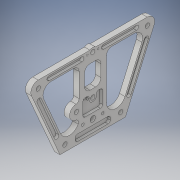
# Autodesk Inventor part: Frame_Bearing
Saved by Autodesk Inventor 2019 (Build 230136000, 136)
## iProperties
Created: 2019-07-29
Part Number: Frame_Bearing
Material: Generic
Document SubType Name: Modeling
Designer: 19879326
Density: 1 g/cm^3
Appearance: Default
Author: 19879326
Autodesk Inventor part; units mm, degrees
ref_plane "YZ Plane" through (0, 0, 0) normal (1, 0, 0) x (0, 1, 0)
ref_plane "XZ Plane" through (0, 0, 0) normal (0, 1, 0) x (-1, 0, 0)
ref_plane "XY Plane" through (0, 0, 0) normal (0, 0, 1) x (1, 0, 0)
sketch "Sketch1" plane through (0, 0, 0) normal (1, 0, 0) x (0, 1, 0)
  line L0 (73.575, 28) -> (65.075, 28)
  line L1 (-73.575, 60) -> (-73.575, -60)
  line L2 (73.575, -28) -> (73.575, 28)
  circle A0 centre (59.575, 0) radius 4
  circle A1 centre (-12.425, 0) radius 4
  circle A2 centre (-46.575, 0) radius 5
  circle A3 centre (-46.575, 18.25) radius 2.5
  circle A4 centre (-46.575, -18.25) radius 2.5
  circle A5 centre (59.575, 0) radius 7.5
  line L3 (65.075, 28) -> (65.075, 5.099)
  line L4 (65.075, -5.099) -> (65.075, -28)
  circle A6 centre (51.575, -100) radius 4
  circle A7 centre (51.575, 100) radius 4
  arc A8 (65.075, 100) -> (46.1655, 112.3688) centre (51.575, 100) ccw
  arc A9 (46.1655, -112.3688) -> (65.075, -100) centre (51.575, -100) ccw
  line L5 (65.075, 28) -> (65.075, 100)
  line L6 (65.075, -28) -> (65.075, -100)
  line L7 (46.1655, 112.3688) -> (-73.575, 60)
  line L8 (-73.575, -60) -> (46.1655, -112.3688)
  line L9 (65.075, -28) -> (73.575, -28)
  line L10 (30.0644, 90.0466) -> (-40.7048, 59.0955)
  line L11 (30.0644, -90.0466) -> (-40.7048, -59.0955)
  line L12 (51.075, 76.3035) -> (51.075, 35)
  line L13 (51.075, -76.3035) -> (51.075, -35)
  line L14 (41.075, 25) -> (-33.575, 25)
  line L15 (41.075, -25) -> (-33.575, -25)
  arc A10 (41.075, 25) -> (51.075, 35) centre (41.075, 35) ccw
  arc A11 (-40.7048, 59.0955) -> (-33.575, 25) centre (-33.575, 42.7932) ccw
  arc A12 (51.075, -35) -> (41.075, -25) centre (41.075, -35) ccw
  line L16 (-31.8814, -25) -> (-33.575, -25)
  arc A13 (-33.575, -25) -> (-40.7048, -59.0955) centre (-33.575, -42.7932) ccw
  line L17 (1.575, 5) -> (1.575, -5)
  arc A14 (43.575, 5) -> (33.575, 15) centre (33.575, 5) ccw
  arc A15 (33.575, -15) -> (43.575, -5) centre (33.575, -5) ccw
  arc A16 (11.575, 15) -> (1.575, 5) centre (11.575, 5) ccw
  arc A17 (1.575, -5) -> (11.575, -15) centre (11.575, -5) ccw
  circle A18 centre (-61.575, 51.0593) radius 4
  circle A19 centre (-61.575, -51.0593) radius 4
  arc A20 (51.075, 76.3035) -> (30.0644, 90.0466) centre (36.075, 76.3035) ccw
  arc A21 (30.0644, -90.0466) -> (51.075, -76.3035) centre (36.075, -76.3035) ccw
  line L18 (43.575, 5) -> (43.575, -5)
  line L19 (33.575, 15) -> (11.575, 15)
  line L20 (33.575, -15) -> (11.575, -15)
  circle A22 centre (-20.425, 30) radius 4
  circle A23 centre (-20.425, 30) radius 12.5
  point P0 (0, 0)
  point P1 (73.575, 0)
  point P2 (51.075, 58.5072)
  point P3 (51.075, -58.5072)
  point P4 (-20.425, -42.5)
  point P5 (16.0532, -25)
  point P6 (-49.2726, -25)
  point P7 (51.075, 59.4738)
  point P8 (43.575, 0)
  point P9 (1.575, 0)
  dimension "d1" = 56
  dimension "d2" = 72
  dimension "d3" = 8
  dimension "d4" = 8
  dimension "d5" = 14
  dimension "d6" = 34.15
  dimension "d7" = 10
  dimension "d8" = 18.25
  dimension "d9" = 18.25
  dimension "d10" = 5
  dimension "d13" = 12.425
  dimension "d14" = 27
  dimension "d15" = 15
  dimension "d18" = 5.5
  dimension "d19" = 8
  dimension "d20" = 100
  dimension "d21" = 100
  dimension "d22" = 8
  dimension "d27" = 60
  dimension "d28" = 60
  dimension "d31" = 14
  dimension "d33" = 14
  dimension "d34" = 14
  dimension "d36" = 25
  dimension "d37" = 25
  dimension "d43" = 40
  dimension "d45" = 14
  dimension "d47" = 12
  dimension "d48" = 13
  dimension "d49" = 13
  dimension "d50" = 12
  dimension "d58" = 10
  dimension "d59" = 15
  dimension "d60" = 16
  dimension "d61" = 10
  dimension "d62" = 10
  dimension "d90" = 8
  dimension "d91" = 25
  dimension "d92" = 30
  dimension "d93" = 8
  constraints: 42 end point, 27 point on circle, 24 centre point, 19 tangent, 12 equal radius, 7 horizontal alignment, 7 point on line, 6 parallel, 6 vertical, 6 vertical alignment, 5 horizontal, 4 coincident, 3 midpoint, 1 perpendicular
  measures "d1" distance of L2.start L0.start
  measures "d2" distance of A1.centre A0.centre
  measures "d3" diameter of A0
  measures "d4" diameter of A1
  measures "d5" distance from line of L2 A0.centre
  measures "d6" distance of A2.centre A1.centre
  measures "d7" diameter of A2
  measures "d8" distance of A3.centre A2.centre
  measures "d9" distance of A4.centre A2.centre
  measures "d10" diameter of A4
  measures "d13" distance of A1.centre point (0, 0)
  measures "d14" distance from line of L1 A2.centre
  measures "d15" diameter of A5
  measures "d18" distance from line of A0.centre L4
  measures "d19" diameter of A7
  measures "d20" vertical distance of A7.centre A0.centre
  measures "d21" vertical distance of A6.centre A0.centre
  measures "d22" horizontal distance of A7.centre A0.centre
  measures "d27" vertical distance of L1.start A2.centre
  measures "d28" vertical distance of L1.end A2.centre
  measures "d31" distance between parallel lines of L5 L12
  measures "d33" distance between parallel lines of L7 L10
  measures "d34" distance between parallel lines of L8 L11
  measures "d36" distance from line of L14 A0.centre
  measures "d37" distance from line of A0.centre L15
  measures "d43" distance from line of L1 A11.centre
  measures "d45" distance from line of A1.centre L17
  measures "d47" distance from line of L1 A18.centre
  measures "d48" distance from line of L7 A18.centre
  measures "d49" distance from line of L8 A19.centre
  measures "d50" distance from line of L1 A19.centre
  measures "d58" radius of A10
  measures "d59" radius of A20
  measures "d60" distance from line of L18 A0.centre
  measures "d61" distance between parallel lines of L15 L20
  measures "d62" distance between parallel lines of L14 L19
  measures "d90" diameter of A22
  measures "d91" diameter of A23
  measures "d92" vertical distance of A22.centre A1.centre
  measures "d93" horizontal distance of A1.centre A22.centre
extrude "Extrusion3" add sketch "Sketch1" along normal blind 10 contours L3 A5 L4 L6 A9 L8 L1 L7 A8 L5 | A5 | A23 L14 | L14 A23
fillet "Fillet1" radius 6 3 edges at (5, -33.575, -25) (5, -31.8814, 25) (5, -8.9686, 25)
sketch "Sketch3" plane through (10, 0, 0) normal (1, 0, 0) x (0, 0, -1)
  line L0 (-18, -36.575) -> (18, -36.575)
  line L1 (18, -36.575) -> (18, -6)
  line L2 (18, -6) -> (-18, -6)
  line L3 (-18, -6) -> (-18, -36.575)
  line L4 (-15, 11.575) -> (-15, 33.575) projected
  line L5 (15, 33.575) -> (15, 11.575) projected
  circle A0 centre (0, -46.575) radius 5 projected
  line L6 (-32.0593, -56.575) -> (32.0593, -56.575)
  line L7 (32.0593, -56.575) -> (32.0593, -68.575)
  line L8 (32.0593, -68.575) -> (-32.0593, -68.575)
  line L9 (-32.0593, -68.575) -> (-32.0593, -56.575)
  line L10 (-60, -73.575) -> (60, -73.575) projected
  line L11 (-102.0122, 29.9722) -> (-70.0199, -43.1778)
  line L12 (-94.6826, 33.1778) -> (-62.6903, -39.9722)
  line L13 (62.6903, -39.9722) -> (94.6826, 33.1778)
  line L14 (90.0466, 30.0644) -> (59.0955, -40.7048) projected
  line L15 (102.0122, 29.9722) -> (70.0199, -43.1778)
  line L16 (60, -73.575) -> (112.3688, 46.1655) projected
  arc A1 (-94.6826, 33.1778) -> (-102.0122, 29.9722) centre (-98.3474, 31.575) ccw
  arc A2 (-70.0199, -43.1778) -> (-62.6903, -39.9722) centre (-66.3551, -41.575) ccw
  arc A3 (102.0122, 29.9722) -> (94.6826, 33.1778) centre (98.3474, 31.575) ccw
  arc A4 (62.6903, -39.9722) -> (70.0199, -43.1778) centre (66.3551, -41.575) ccw
  line L17 (-59.0955, -40.7048) -> (-90.0466, 30.0644) projected
  line L18 (-112.3688, 46.1655) -> (-60, -73.575) projected
  line L19 (-80, 62.075) -> (-20, 62.075)
  line L20 (-20, 54.075) -> (-80, 54.075)
  line L21 (20, 62.075) -> (80, 62.075)
  line L22 (80, 54.075) -> (20, 54.075)
  arc A5 (-80, 62.075) -> (-80, 54.075) centre (-80, 58.075) ccw
  arc A6 (-20, 54.075) -> (-20, 62.075) centre (-20, 58.075) ccw
  arc A7 (20, 62.075) -> (20, 54.075) centre (20, 58.075) ccw
  arc A8 (80, 54.075) -> (80, 62.075) centre (80, 58.075) ccw
  circle A9 centre (0, 59.575) radius 4 projected
  line L23 (-5.099, 65.075) -> (-100, 65.075) projected
  line L24 (-76.3035, 51.075) -> (-35, 51.075) projected
  line L25 (35, 51.075) -> (76.3035, 51.075) projected
  line L26 (100, 65.075) -> (5.099, 65.075) projected
  circle A10 centre (0, -12.425) radius 7
  circle A11 centre (0, -12.425) radius 4 projected
  circle A12 centre (-100, 51.575) radius 4
  circle A13 centre (100, 51.575) radius 4
  circle A14 centre (-51.0593, -61.575) radius 4 projected
  circle A15 centre (-51.0593, -61.575) radius 4
  circle A16 centre (-100, 51.575) radius 4 projected
  circle A17 centre (100, 51.575) radius 4 projected
  circle A18 centre (-51.0593, -61.575) radius 4 projected
  point P0 (0, 0)
  dimension "d63" = 3
  dimension "d64" = 3
  dimension "d65" = 6
  dimension "d66" = 10
  dimension "d67" = 5
  dimension "d68" = 10
  dimension "d71" = 3
  dimension "d72" = 3
  dimension "d73" = 3
  dimension "d74" = 3
  dimension "d78" = 20
  dimension "d79" = 20
  dimension "d81" = 3
  dimension "d82" = 3
  dimension "d83" = 3
  dimension "d84" = 3
  dimension "d87" = 14
  dimension "d113" = 20
  dimension "d114" = 20
  dimension "d115" = 20
  dimension "d117" = 20
  constraints: 32 end point, 16 point on circle, 16 tangent, 12 centre point, 10 parallel, 7 concentric, 4 horizontal, 3 perpendicular, 2 horizontal alignment
  measures "d63" distance between parallel lines of L4 L3
  measures "d64" distance between parallel lines of L1 L5
  measures "d65" distance from line of L2 point (0, 0)
  measures "d66" distance from line of A0.centre L0
  measures "d67" distance between parallel lines of L8 L10
  measures "d68" distance from line of L6 A0.centre
  measures "d71" distance between parallel lines of L17 L12
  measures "d72" distance between parallel lines of L18 L11
  measures "d73" distance between parallel lines of L16 L15
  measures "d74" distance between parallel lines of L14 L13
  measures "d78" horizontal distance of A9.centre A6.centre
  measures "d79" horizontal distance of A7.centre A9.centre
  measures "d81" distance between parallel lines of L23 L19
  measures "d82" distance between parallel lines of L24 L20
  measures "d83" distance between parallel lines of L25 L22
  measures "d84" distance between parallel lines of L26 L21
  measures "d87" diameter of A10
  measures "d113" horizontal distance of A12.centre A5.centre
  measures "d114" vertical distance of A1.centre A16.centre
  measures "d115" horizontal distance of A8.centre A13.centre
  measures "d117" vertical distance of A2.centre A15.centre
extrude "Extrusion5" cut sketch "Sketch3" against normal blind 5 contours L3 L2 A10 L1 L0 | L6 L7 L8 L9 | A1 L12 A2 L11 | L13 A3 L15 A4 | L19 A6 L20 A5 | L21 A8 L22 A7
fillet "Fillet2" radius 4 10 edges at (7.5, -6, 18) (7.5, -36.575, 18) (7.5, -36.575, -18) (7.5, -6, -18) (7.5, -6, 2.7784) (7.5, -6, -2.7784) (7.5, -56.575, 32.0593) (7.5, -56.575, -32.0593) (7.5, -68.575, -32.0593) (7.5, -68.575, 32.0593)
sketch "Sketch4" plane through (10, -32.6529, 0.9304) normal (1, 0, 0) x (0, 0, -1)
  circle A0 centre (-9.0696, 92.2279) radius 1.5
  circle A1 centre (10.9304, 92.2279) radius 1.5
  circle A2 centre (0.9304, 92.2279) radius 4
  circle A3 centre (0.9304, 92.2279) radius 4
  circle A4 centre (0.9304, 92.2279) radius 4 projected
  circle A5 centre (-9.0696, 20.2279) radius 1.5
  circle A6 centre (10.9304, 20.2279) radius 1.5
  circle A7 centre (0.9304, 20.2279) radius 4
  circle A8 centre (0.9304, 20.2279) radius 4
  circle A9 centre (0.9304, 20.2279) radius 4
  circle A10 centre (0.9304, 20.2279) radius 4 projected
  circle A11 centre (-9.0696, 20.2279) radius 1.5
  circle A12 centre (10.9304, 20.2279) radius 1.5
  point P0 (0, 0)
  dimension "d106" = 3
  dimension "d105" = 10
  dimension "d104" = 10
  dimension "d110" = 3
  dimension "d111" = 10
  dimension "d112" = 10
  constraints: 11 centre point, 9 equal radius, 5 concentric, 4 horizontal alignment, 2 coincident
  measures "d106" diameter of A0
  measures "d105" distance of A2.centre A0.centre
  measures "d104" distance of A1.centre A2.centre
  measures "d110" diameter of A5
  measures "d111" distance of A7.centre A5.centre
  measures "d112" distance of A6.centre A7.centre
extrude "Extrusion6" cut sketch "Sketch4" against normal blind 10 contours A0 | A1 | A5 | A6
body "Solid3"
